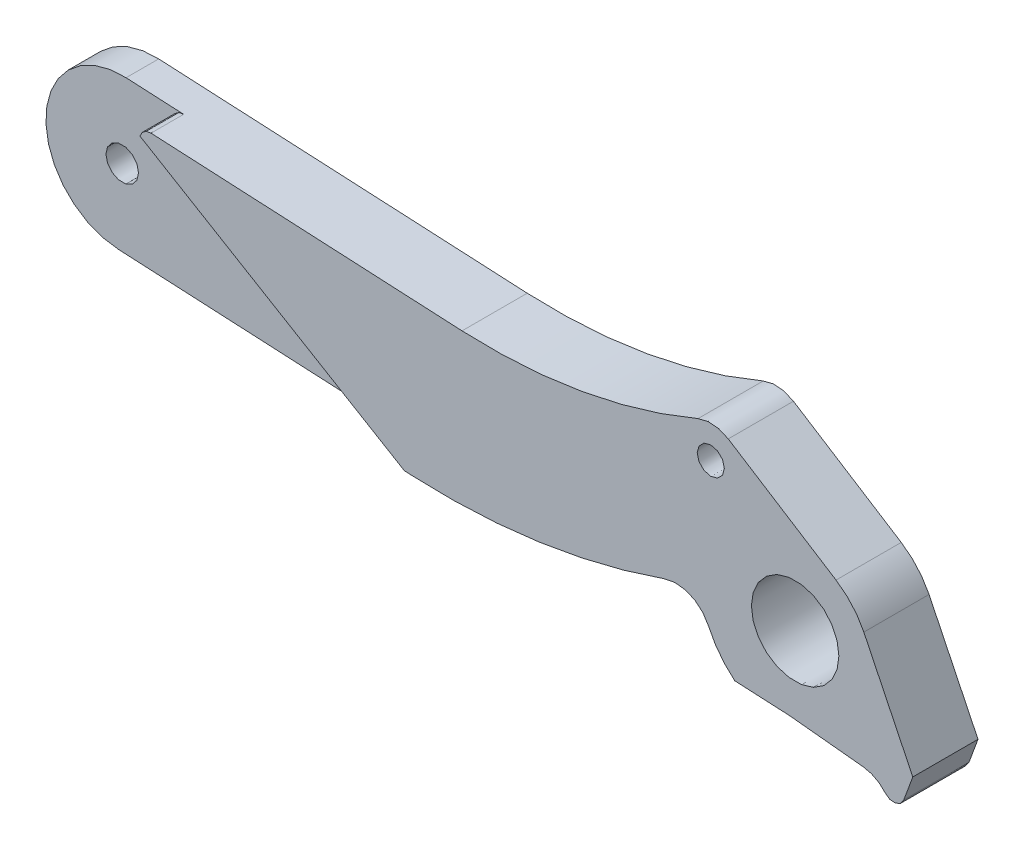
# Autodesk Inventor part: 後ろウイング根本
Saved by Autodesk Inventor 2020 (Build 240168000, 168)
## iProperties
Created: 2019-12-28
Part Number: 後ろウイング根本
Material: ポリカーボネート、クリア
Document SubType Name: Modeling
Designer: tanjihayato
Density: 1.2 g/cm^3
Appearance: ポリカーボネート - クリア
Author: tanjihayato
Autodesk Inventor part; units mm, degrees
ref_plane "YZ Plane" through (0, 0, 0) normal (1, 0, 0) x (0, 1, 0)
ref_plane "XZ Plane" through (0, 0, 0) normal (0, 1, 0) x (-1, 0, 0)
ref_plane "XY Plane" through (0, 0, 0) normal (0, 0, 1) x (1, 0, 0)
sketch "スケッチ1" plane through (0, 0, 0) normal (0, 0, 1) x (1, 0, 0)
  circle A0 centre (-145.5257, 0.5882) radius 1.5
  circle A1 centre (-139.5445, -10.0968) radius 1.5
  circle A2 centre (-105.5257, -16.4118) radius 30.1 construction
  line L0 (-170.915, -81.4118) -> (490.0044, -81.4118)
  circle A3 centre (-145.5257, 0.5882) radius 4.025
  circle A4 centre (-139.5445, -10.0968) radius 3
  circle A5 centre (-145.5257, 0.5882) radius 7.025
  line L1 (-146.2365, -6.4007) -> (-139.241, -7.1122)
  line L2 (-139.2044, 3.6529) -> (-134.6999, -5.6381)
  line L3 (-134.6999, -5.6381) -> (-136.7303, -11.1361)
  circle A6 centre (-105.5257, -16.4118) radius 31.1 construction
  line L4 (-145.1707, 7.6042) -> (-210.0877, 10.8882)
  line L5 (-145.8806, -6.4278) -> (-210.7976, -3.1438)
  circle A7 centre (-210.4427, 3.8722) radius 1.5
  circle A8 centre (-210.4427, 3.8722) radius 4.025
  circle A9 centre (-210.4427, 3.8722) radius 7.025
  circle A10 centre (-210.4427, 3.8722) radius 7.525
  line L6 (-206.5907, 10.3366) -> (-181.4786, -4.627)
  circle A11 centre (-199.4194, 13.3524) radius 1.25
  arc A12 (-199.5709, 10.3562) -> (-202.1936, 14.494) centre (-199.4194, 13.3524) ccw
  line L7 (-202.1936, 14.494) -> (-247.2482, 16.7732)
  arc A13 (-289.8377, 39.1951) -> (-247.2482, 16.7732) centre (-244.3571, 73.9244) ccw
  arc A14 (-289.8377, 39.1951) -> (-291.5649, 38.2266) centre (-290.6325, 38.5882) ccw
  arc A15 (-291.5649, 38.2266) -> (-251.8636, 4.9117) centre (-241.4172, 57.674) ccw
  line L8 (-251.8636, 4.9117) -> (-211.807, -3.019)
  line L9 (-209.3045, 11.3106) -> (-204.7936, 10.6204)
  arc A16 (-204.7936, 10.6204) -> (-205.5417, 8.9052) centre (-204.8441, 9.6217) ccw
  line L10 (-210.5022, 11.397) -> (-238.3358, 2.2334)
  point P0 (0, 0)
  point P1 (0, 0)
  point P2 (-146.0589, -6.4188)
  point P3 (-205.8121, 9.8726)
  dimension "d0" = 6
  dimension "d1" = 8.05
  dimension "d2" = 3
  dimension "d3" = 1
  dimension "d4" = 3
  dimension "d5" = 8.05
  dimension "d6" = 3
  dimension "d7" = 0.5
  dimension "d8" = 2.5
  dimension "d9" = 6
  dimension "d10" = 2
  dimension "d11" = 120
  dimension "d12" = 4
  dimension "d13" = 150
  dimension "d14" = 1
  dimension "d15" = 65
  dimension "d16" = 87.382
  constraints: 23 point on circle, 22 end point, 18 tangent, 16 centre point, 4 coincident, 4 point on line, 1 parallel, 6 other
  measures "d0" diameter of A4
  measures "d1" diameter of A3
  measures "d2" radial gap between concentric circles of A3 A5
  measures "d4" diameter of A7
  measures "d5" diameter of A8
  measures "d6" radial gap between concentric circles of A8 A9
  measures "d7" radial gap between concentric circles of A9 A10
  measures "d8" diameter of A11
  measures "d9" diameter of A12
  measures "d10" diameter of A14
  measures "d11" distance from line of L0 A14.centre
  measures "d12" distance between parallel lines of L4 L7
  measures "d13" distance of A14.centre A0.centre
  measures "d14" radius of A16
  measures "d15" distance of A0.centre A7.centre
  measures "d16" distance of A14.centre A7.centre
extrude "押し出し1" add sketch "スケッチ1" along normal blind 6 contours A4 L1 L5 A5 L2 L3 | L5 L6 A16 L4 A5 L1 | A5
extrude "押し出し2" add sketch "スケッチ1" along normal blind 3 contours L5 A10 A16 L6 | L5 A9 A16 A10 | A16 A10 L6 | L6 A10 L4 A16 | A9 | A10 A16 A9 L4 | A8
fillet "フィレット1" radius 1 1 edges at (-136.7303, -11.1361, 3)
sketch "スケッチ2" plane through (0, 0, 6) normal (0, 0, 1) x (1, 0, 0)
  line L0 (-210.7976, -3.1438) -> (-181.4786, -4.627) projected
  line L1 (-205.8121, 9.8726) -> (-181.4786, -4.627) projected
  arc A0 (-204.7936, 10.6204) -> (-205.8121, 9.8726) centre (-204.8441, 9.6217) ccw projected
  line L2 (-204.7936, 10.6204) -> (-210.0877, 10.8882) projected
  arc A1 (-210.0877, 10.8882) -> (-210.7976, -3.1438) centre (-210.4427, 3.8722) ccw projected
  circle A2 centre (-210.4427, 3.8722) radius 1.5 projected
  arc A3 (-137.2374, -8.1793) -> (-135.5302, -7.8865) centre (-136.4683, -7.5401) ccw projected
  line L3 (-135.5302, -7.8865) -> (-134.6999, -5.6381) projected
  line L4 (-134.6999, -5.6381) -> (-139.2044, 3.6529) projected
  arc A4 (-139.2044, 3.6529) -> (-145.1707, 7.6042) centre (-145.5257, 0.5882) ccw projected
  line L5 (-145.1707, 7.6042) -> (-204.7936, 10.6204) projected
  arc A5 (-204.7936, 10.6204) -> (-205.8121, 9.8726) centre (-204.8441, 9.6217) ccw projected
  line L6 (-205.8121, 9.8726) -> (-181.4786, -4.627) projected
  line L7 (-181.4786, -4.627) -> (-146.0589, -6.4188) projected
  line L8 (-146.0589, -6.4188) -> (-146.2365, -6.4007) projected
  arc A6 (-146.2365, -6.4007) -> (-145.8806, -6.4278) centre (-145.5257, 0.5882) ccw projected
  line L9 (-145.8806, -6.4278) -> (-146.0589, -6.4188) projected
  line L10 (-146.0589, -6.4188) -> (-139.241, -7.1122) projected
  arc A7 (-137.2374, -8.1793) -> (-139.241, -7.1122) centre (-139.5445, -10.0968) ccw projected
  circle A8 centre (-145.5257, 0.5882) radius 4.025 projected
  arc A9 (-204.7936, 10.6204) -> (-205.8121, 9.8726) centre (-204.8441, 9.6217) ccw projected
  line L11 (-204.6925, 12.6179) -> (-209.9867, 12.8857)
  arc A10 (-209.9867, 12.8857) -> (-210.8986, -5.1413) centre (-210.4427, 3.8722) ccw
  arc A11 (-182.0757, -6.5994) -> (-181.4786, -4.627) centre (-182.022, -5.539) ccw
  line L12 (-210.8986, -5.1413) -> (-182.0757, -6.5994)
  arc A12 (-204.7936, 10.6204) -> (-204.6925, 12.6179) centre (-204.743, 11.6191) ccw
  point P0 (0, 0)
  dimension "d22" = 2
  constraints: 6 point on circle, 6 tangent, 4 end point, 3 centre point, 2 parallel, 1 coincident
  measures "d22" distance between parallel lines of L12 L0
sketch "スケッチ3" plane through (0, 0, 6) normal (0, 0, 1) x (1, 0, 0)
  arc A0 (-137.2374, -8.1793) -> (-135.5302, -7.8865) centre (-136.4683, -7.5401) ccw projected
  line L0 (-135.5302, -7.8865) -> (-134.6999, -5.6381) projected
  line L1 (-134.6999, -5.6381) -> (-139.2044, 3.6529) projected
  arc A1 (-139.2044, 3.6529) -> (-145.1707, 7.6042) centre (-145.5257, 0.5882) ccw projected
  line L2 (-145.1707, 7.6042) -> (-204.7936, 10.6204) projected
  arc A2 (-204.7936, 10.6204) -> (-205.8121, 9.8726) centre (-204.8441, 9.6217) ccw projected
  line L3 (-205.8121, 9.8726) -> (-181.4786, -4.627) projected
  line L4 (-181.4786, -4.627) -> (-146.0589, -6.4188) projected
  line L5 (-146.0589, -6.4188) -> (-146.2365, -6.4007) projected
  arc A3 (-146.2365, -6.4007) -> (-145.8806, -6.4278) centre (-145.5257, 0.5882) ccw projected
  line L6 (-145.8806, -6.4278) -> (-146.0589, -6.4188) projected
  line L7 (-146.0589, -6.4188) -> (-139.241, -7.1122) projected
  arc A4 (-137.2374, -8.1793) -> (-139.241, -7.1122) centre (-139.5445, -10.0968) ccw projected
  circle A5 centre (-145.5257, 0.5882) radius 4.025 projected
  point P0 (0, 0)
extrude "押し出し3" add sketch "スケッチ3" against normal blind 6 contours L5 A3 L6
sketch "スケッチ4" plane through (0, 0, 6) normal (0, 0, 1) x (1, 0, 0)
  line L0 (-146.0589, -6.4188) -> (-139.241, -7.1122) projected
  arc A0 (-137.2374, -8.1793) -> (-139.241, -7.1122) centre (-139.5445, -10.0968) ccw projected
  arc A1 (-137.2374, -8.1793) -> (-135.5302, -7.8865) centre (-136.4683, -7.5401) ccw projected
  line L1 (-135.5302, -7.8865) -> (-134.6999, -5.6381) projected
  line L2 (-134.6999, -5.6381) -> (-139.2044, 3.6529) projected
  arc A2 (-139.2044, 3.6529) -> (-145.1707, 7.6042) centre (-145.5257, 0.5882) ccw projected
  line L3 (-145.1707, 7.6042) -> (-204.7936, 10.6204) projected
  arc A3 (-204.7936, 10.6204) -> (-205.8121, 9.8726) centre (-204.8441, 9.6217) ccw projected
  line L4 (-205.8121, 9.8726) -> (-181.4786, -4.627) projected
  line L5 (-181.4786, -4.627) -> (-146.0589, -6.4188) projected
  circle A4 centre (-145.5257, 0.5882) radius 4.025 projected
  arc A5 (-153.4999, -3.002) -> (-157.5446, -1.2714) centre (-156.4634, -4.3363) ccw
  arc A6 (-180.854, -4.6586) -> (-157.5446, -1.2714) centre (-177.7808, 56.0903) ccw
  line L6 (-181.4786, -4.627) -> (-146.0589, -6.4188) projected
  circle A7 centre (-139.5445, -10.0968) radius 3 projected
  arc A8 (-153.4999, -3.002) -> (-151.0823, -6.1647) centre (-145.5257, 0.5882) ccw
  line L7 (-145.1707, 7.6042) -> (-204.7936, 10.6204) projected
  arc A9 (-176.1768, 9.1728) -> (-154.4643, 13.0367) centre (-173.6978, 58.1782) ccw
  arc A10 (-151.6818, 12.8103) -> (-154.4643, 13.0367) centre (-153.2884, 10.2768) ccw
  line L8 (-151.6818, 12.8103) -> (-141.7636, 6.5209)
  circle A11 centre (-153.2884, 10.2768) radius 1.25
  circle A12 centre (-139.5445, -10.0968) radius 3.5
  point P0 (0, 0)
  point P1 (-176.1768, 9.1728)
  dimension "d25" = 3.25
  dimension "d26" = 95
  dimension "d27" = 3
  dimension "d28" = 2.5
  dimension "d29" = 0.5
  constraints: 11 point on circle, 8 tangent, 7 centre point, 3 point on line, 2 coincident, 2 end point
  measures "d25" radius of A5
  measures "d27" radius of A10
  measures "d28" diameter of A11
  measures "d29" radial gap between concentric circles of A12 A7
extrude "押し出し4" cut sketch "スケッチ4" against normal blind 6 contours L5 A6 A5 A8
extrude "押し出し5" add sketch "スケッチ4" against normal blind 6 contours A2 L3 A9 A10 L8
sketch "スケッチ5" plane through (0, 0, 6) normal (0, 0, 1) x (1, 0, 0)
  circle A0 centre (-153.2884, 10.2768) radius 1.25 projected
  circle A1 centre (-145.5257, 0.5882) radius 4.025 projected
  arc A2 (-180.854, -4.6586) -> (-157.5446, -1.2714) centre (-177.7808, 56.0903) ccw projected
  arc A3 (-153.4999, -3.002) -> (-157.5446, -1.2714) centre (-156.4634, -4.3363) ccw projected
  arc A4 (-153.4999, -3.002) -> (-151.0823, -6.1647) centre (-145.5257, 0.5882) ccw projected
  line L0 (-151.0823, -6.1647) -> (-146.0589, -6.4188) projected
  line L1 (-146.0589, -6.4188) -> (-139.241, -7.1122) projected
  arc A5 (-137.2374, -8.1793) -> (-139.241, -7.1122) centre (-139.5445, -10.0968) ccw projected
  arc A6 (-137.2374, -8.1793) -> (-135.5302, -7.8865) centre (-136.4683, -7.5401) ccw projected
  line L2 (-135.5302, -7.8865) -> (-134.6999, -5.6381) projected
  line L3 (-134.6999, -5.6381) -> (-139.2044, 3.6529) projected
  arc A7 (-139.2044, 3.6529) -> (-141.7636, 6.5209) centre (-145.5257, 0.5882) ccw projected
  line L4 (-141.7636, 6.5209) -> (-151.6818, 12.8103) projected
  arc A8 (-151.6818, 12.8103) -> (-154.4643, 13.0367) centre (-153.2884, 10.2768) ccw projected
  arc A9 (-176.1768, 9.1728) -> (-154.4643, 13.0367) centre (-173.6978, 58.1782) ccw projected
  line L5 (-176.1768, 9.1728) -> (-204.7936, 10.6204) projected
  arc A10 (-204.7936, 10.6204) -> (-205.8121, 9.8726) centre (-204.8441, 9.6217) ccw projected
  line L6 (-205.8121, 9.8726) -> (-181.4786, -4.627) projected
  line L7 (-181.4786, -4.627) -> (-180.854, -4.6586) projected
  line L8 (-204.7936, 10.6204) -> (-210.0877, 10.8882) projected
  arc A11 (-210.0877, 10.8882) -> (-210.7976, -3.1438) centre (-210.4427, 3.8722) ccw projected
  line L9 (-210.7976, -3.1438) -> (-181.4786, -4.627) projected
  line L10 (-205.8121, 9.8726) -> (-181.4786, -4.627) projected
  arc A12 (-204.7936, 10.6204) -> (-205.8121, 9.8726) centre (-204.8441, 9.6217) ccw projected
  circle A13 centre (-210.4427, 3.8722) radius 1.5 projected
  arc A14 (-204.7936, 10.6204) -> (-205.8121, 9.8726) centre (-204.8441, 9.6217) ccw projected
  arc A15 (-204.7936, 10.6204) -> (-204.6925, 12.6179) centre (-204.743, 11.6191) ccw
  line L11 (-204.6925, 12.6179) -> (-209.9867, 12.8857)
  arc A16 (-209.9867, 12.8857) -> (-210.8986, -5.1413) centre (-210.4427, 3.8722) ccw
  line L12 (-210.8986, -5.1413) -> (-182.0757, -6.5994)
  arc A17 (-182.0757, -6.5994) -> (-181.4786, -4.627) centre (-182.022, -5.539) ccw
  line L13 (-205.8121, 9.8726) -> (-181.4786, -4.627) projected
  point P0 (0, 0)
  dimension "d34" = 2
  constraints: 6 point on circle, 6 tangent, 4 end point, 3 centre point, 2 parallel, 1 coincident
  measures "d34" radial gap between concentric circles of A16 A11
